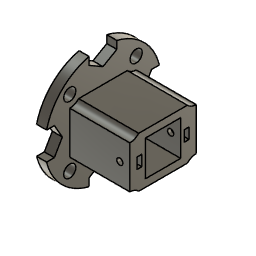
Main_Shredder (Autodesk Fusion 360 archive; units mm, degrees)
design "GearBox_Axle_Conector"
Autodesk Fusion 360 part; units mm, degrees
sketch "Plate" plane through (0, 0, 0) normal (0, 0, 1) x (1, 0, 0)
  circle A0 centre (-28.284, 0) radius 11
  line L0 (0, 0) -> (-28.284, 0) construction
  circle A1 centre (-28.284, 0) radius 4.05
  circle A2 centre (0, -28.284) radius 4.05
  circle A3 centre (0, -28.284) radius 11
  circle A4 centre (28.284, 0) radius 4.05
  circle A5 centre (28.284, 0) radius 11
  circle A6 centre (0, 28.284) radius 4.05
  circle A7 centre (0, 28.284) radius 11
  circle A8 centre (0, 0) radius 39
  dimension "d2" = 22
  dimension "d8" = 28.284
  dimension "d9" = 8.1
  dimension "d11" = 360
  dimension "d42" = 78
  constraint coincident L0.start A8.centre
  constraint coincident A0.centre L0.end
  constraint horizontal L0
  constraint concentric A0 A1
  measures "d2" diameter of A0
  measures "d8" distance of L0.start A0.centre
  measures "d9" diameter of A1
  measures "d42" diameter of A8
extrude "Extrude1" add sketch "Plate" along normal blind 3 contours A0 A8 | A0 A8 | A7 A8 | A7 A8 | A3 A8 | A3 A8 | A5 A8 | A5 A8 makes body 1 at (8.6273, 27.5363, 0) makes body 2 at (36.9113, 0.7477, 3) makes body 3 at (-19.6416, 0.5465, 3) makes body 4 at (8.6273, -27.5363, 3)
extrude "Extrude2" add sketch "Plate" against normal blind 13 bodies 1 2 3 4
chamfer "Chamfer1" distance 5.5 distance2 2.5 4 edges at (-10.2556, 24.3062, 3) (-38.5396, -3.9778, 3) (-10.2556, -32.2618, 3) (18.0284, -3.9778, 3) measured on face at (8.6424, 28.8305, 3) measured on face at (-19.6416, 0.5465, 3) measured on face at (8.6273, -27.5363, 3) measured on face at (36.9113, 0.7477, 3) on bodies 1
extrude "Extrude9" add 4 faces at (-23.2878, 0.2732, 3) (33.2802, 0.2732, 3) (4.9962, 28.5572, 3) (4.9962, -28.0108, 3) along direction (0, 0, 1) blind 1.2 on bodies 1 bodies 1
sketch "BallbearingHole" plane through (0, 0, 0) normal (0, 0, 1) x (1, 0, 0)
  arc A0 (-38.891, -2.9141) -> (-38.891, 2.9141) centre (-28.284, 0) ccw
  arc A1 (-38.891, -2.9141) -> (-2.9141, -38.891) centre (0, 0) ccw
  arc A2 (2.9141, -38.891) -> (-2.9141, -38.891) centre (0, -28.284) ccw
  arc A3 (2.9141, -38.891) -> (38.891, -2.9141) centre (0, 0) ccw
  arc A4 (38.891, 2.9141) -> (38.891, -2.9141) centre (28.284, 0) ccw
  arc A5 (38.891, 2.9141) -> (2.9141, 38.891) centre (0, 0) ccw
  arc A6 (-2.9141, 38.891) -> (2.9141, 38.891) centre (0, 28.284) ccw
  arc A7 (-2.9141, 38.891) -> (-38.891, 2.9141) centre (0, 0) ccw
  circle A8 centre (0, 0) radius 16
  dimension "d22" = 32
  constraint coincident A1.centre A3.centre
  measures "d22" diameter of A8
extrude "Extrude3" cut sketch "BallbearingHole" against normal blind 9.5 contours A8 bodies 1
sketch "BallbearingStandoff" plane through (0, 0, -9.5) normal (0, 0, 1) x (1, 0, 0)
  circle A0 centre (0, 0) radius 16
  circle A1 centre (0, 0) radius 15
  dimension "d25" = -1
extrude "Extrude4" add sketch "BallbearingStandoff" along normal blind 0.5 bodies 1
sketch "Nut" plane through (0, 0, -13) normal (0, 0, -1) x (-1, 0, 0)
  circle A0 centre (-28.284, 0) radius 4.05
  circle A1 centre (0, -28.284) radius 4.05
  circle A2 centre (28.284, 0) radius 4.05
  circle A3 centre (0, 28.284) radius 4.05
  arc A4 (-38.891, 2.9141) -> (-38.891, -2.9141) centre (-28.284, 0) ccw
  arc A5 (-38.891, -2.9141) -> (-2.9141, -38.891) centre (0, 0) ccw
  arc A6 (-2.9141, -38.891) -> (2.9141, -38.891) centre (0, -28.284) ccw
  arc A7 (2.9141, -38.891) -> (38.891, -2.9141) centre (0, 0) ccw
  arc A8 (38.891, -2.9141) -> (38.891, 2.9141) centre (28.284, 0) ccw
  arc A9 (38.891, 2.9141) -> (2.9141, 38.891) centre (0, 0) ccw
  arc A10 (2.9141, 38.891) -> (-2.9141, 38.891) centre (0, 28.284) ccw
  arc A11 (-2.9141, 38.891) -> (-38.891, 2.9141) centre (0, 0) ccw
  line L0 (-32.284, -6.9282) -> (-36.284, 0)
  line L1 (-36.284, 0) -> (-32.284, 6.9282)
  line L2 (-32.284, 6.9282) -> (-24.284, 6.9282)
  line L3 (-24.284, 6.9282) -> (-20.284, 0)
  line L4 (-20.284, 0) -> (-24.284, -6.9282)
  line L5 (-24.284, -6.9282) -> (-32.284, -6.9282)
  line L6 (-20.284, 0) -> (-36.284, 0) construction
  line L7 (-6.9282, -24.284) -> (0, -20.284)
  line L8 (-6.9282, -32.284) -> (-6.9282, -24.284)
  line L9 (0, -36.284) -> (-6.9282, -32.284)
  line L10 (6.9282, -32.284) -> (0, -36.284)
  line L11 (6.9282, -24.284) -> (6.9282, -32.284)
  line L12 (0, -20.284) -> (6.9282, -24.284)
  line L13 (24.284, -6.9282) -> (20.284, 0)
  line L14 (32.284, -6.9282) -> (24.284, -6.9282)
  line L15 (36.284, 0) -> (32.284, -6.9282)
  line L16 (32.284, 6.9282) -> (36.284, 0)
  line L17 (24.284, 6.9282) -> (32.284, 6.9282)
  line L18 (20.284, 0) -> (24.284, 6.9282)
  line L19 (6.9282, 24.284) -> (0, 20.284)
  line L20 (6.9282, 32.284) -> (6.9282, 24.284)
  line L21 (0, 36.284) -> (6.9282, 32.284)
  line L22 (-6.9282, 32.284) -> (0, 36.284)
  line L23 (-6.9282, 24.284) -> (-6.9282, 32.284)
  line L24 (0, 20.284) -> (-6.9282, 24.284)
  dimension "d28" = 120
  dimension "d29" = 120
  dimension "d30" = 120
  dimension "d31" = 8
  dimension "d33" = 360
  constraint equal L0 L1
  constraint equal L1 L2
  constraint equal L2 L3
  constraint equal L3 L4
  constraint equal L4 L5
  constraint horizontal L6
  constraint midpoint A0.centre L6
  measures "d28" angle of L0 L1
  measures "d29" angle of L1 L2
  measures "d30" angle of L2 L3
  measures "d31" distance of L0.end L1.end
  measures "d70" distance of L16.start
  measures "d71" distance of L16.start
extrude "Extrude5" cut sketch "Nut" against normal blind 11.5 contours L0 L1 L2 L3 L4 L5 | L7 L8 L9 L10 L11 L12 | L13 L14 L15 L16 L17 L18 | L19 L20 L21 L22 L23 L24 bodies 1
sketch "Output" plane through (0, 0, -13) normal (0, 0, -1) x (-1, 0, 0)
  line L0 (-24.284, 6.9282) -> (-20.284, 0)
  line L1 (-20.284, 0) -> (-24.284, -6.9282)
  line L2 (-24.284, -6.9282) -> (-32.284, -6.9282)
  line L3 (-32.284, -6.9282) -> (-36.284, 0)
  line L4 (-36.284, 0) -> (-32.284, 6.9282)
  line L5 (-32.284, 6.9282) -> (-24.284, 6.9282)
  line L6 (32.284, -6.9282) -> (24.284, -6.9282)
  line L7 (24.284, -6.9282) -> (20.284, 0)
  line L8 (20.284, 0) -> (24.284, 6.9282)
  line L9 (24.284, 6.9282) -> (32.284, 6.9282)
  line L10 (32.284, 6.9282) -> (36.284, 0)
  line L11 (36.284, 0) -> (32.284, -6.9282)
  line L12 (6.9282, 32.284) -> (6.9282, 24.284)
  line L13 (6.9282, 24.284) -> (0, 20.284)
  line L14 (0, 20.284) -> (-6.9282, 24.284)
  line L15 (-6.9282, 24.284) -> (-6.9282, 32.284)
  line L16 (-6.9282, 32.284) -> (0, 36.284)
  line L17 (0, 36.284) -> (6.9282, 32.284)
  line L18 (-6.9282, -32.284) -> (-6.9282, -24.284)
  line L19 (-6.9282, -24.284) -> (0, -20.284)
  line L20 (0, -20.284) -> (6.9282, -24.284)
  line L21 (6.9282, -24.284) -> (6.9282, -32.284)
  line L22 (6.9282, -32.284) -> (0, -36.284)
  line L23 (0, -36.284) -> (-6.9282, -32.284)
  arc A0 (-38.891, 2.9141) -> (-38.891, -2.9141) centre (-28.284, 0) ccw
  arc A1 (-38.891, -2.9141) -> (-2.9141, -38.891) centre (0, 0) ccw
  arc A2 (-2.9141, -38.891) -> (2.9141, -38.891) centre (0, -28.284) ccw
  arc A3 (2.9141, -38.891) -> (38.891, -2.9141) centre (0, 0) ccw
  arc A4 (38.891, -2.9141) -> (38.891, 2.9141) centre (28.284, 0) ccw
  arc A5 (38.891, 2.9141) -> (2.9141, 38.891) centre (0, 0) ccw
  arc A6 (2.9141, 38.891) -> (-2.9141, 38.891) centre (0, 28.284) ccw
  arc A7 (-2.9141, 38.891) -> (-38.891, 2.9141) centre (0, 0) ccw
  circle A8 centre (0, 0) radius 30
  dimension "d39" = 60
  constraint concentric A1 A8
  measures "d39" diameter of A8
extrude "Extrude6" add sketch "Output" along normal blind 13 contours L0 L1 L2 L5 L6 L7 L8 L9 L12 L13 L14 L15 L18 L19 L20 L21 A8 bodies 1
sketch "Mounting hole Output" plane through (0, 0, -26) normal (0, 0, -1) x (-1, 0, 0)
  line L0 (24.284, 6.9282) -> (29.189, 6.9282)
  arc A0 (29.189, 6.9282) -> (6.9282, 29.189) centre (0, 0) ccw
  line L1 (6.9282, 29.189) -> (6.9282, 24.284)
  line L2 (6.9282, 24.284) -> (0, 20.284)
  line L3 (0, 20.284) -> (-6.9282, 24.284)
  line L4 (-6.9282, 24.284) -> (-6.9282, 29.189)
  arc A1 (-6.9282, 29.189) -> (-29.189, 6.9282) centre (0, 0) ccw
  line L5 (-29.189, 6.9282) -> (-24.284, 6.9282)
  line L6 (-24.284, 6.9282) -> (-20.284, 0)
  line L7 (-20.284, 0) -> (-24.284, -6.9282)
  line L8 (-24.284, -6.9282) -> (-29.189, -6.9282)
  arc A2 (-29.189, -6.9282) -> (-6.9282, -29.189) centre (0, 0) ccw
  line L9 (-6.9282, -29.189) -> (-6.9282, -24.284)
  line L10 (-6.9282, -24.284) -> (0, -20.284)
  line L11 (0, -20.284) -> (6.9282, -24.284)
  line L12 (6.9282, -24.284) -> (6.9282, -29.189)
  arc A3 (6.9282, -29.189) -> (29.189, -6.9282) centre (0, 0) ccw
  line L13 (29.189, -6.9282) -> (24.284, -6.9282)
  line L14 (24.284, -6.9282) -> (20.284, 0)
  line L15 (20.284, 0) -> (24.284, 6.9282)
  circle A4 centre (-16.5817, 16.5817) radius 3.05
  line L16 (0, 0) -> (-16.5817, 16.5817) construction
  line L17 (0, 0) -> (-16.5817, 0) construction
  line L18 (-16.5817, 0) -> (-16.5817, 16.5817) construction
  circle A5 centre (-16.5817, -16.5817) radius 3.05
  circle A6 centre (16.5817, -16.5817) radius 3.05
  circle A7 centre (16.5817, 16.5817) radius 3.05
  dimension "d44" = 6.1
  dimension "d45" = 23.45
  dimension "d47" = 360
  constraint coincident A0.centre A1.centre
  constraint coincident A4.centre L16.end
  constraint horizontal L17
  constraint vertical L18
  constraint equal L17 L18
  measures "d44" diameter of A4
  measures "d45" distance of A0.centre A4.centre
extrude "Extrude7" cut sketch "Mounting hole Output" against normal blind 24.5 contours A4 | A5 | A6 | A7 bodies 1
sketch "OutputHub Nut" plane through (0, 0, 0) normal (0, 0, 1) x (1, 0, 0)
  circle A0 centre (0, 0) radius 16
  arc A1 (-38.891, -2.9141) -> (-38.891, 2.9141) centre (-28.284, 0) ccw
  arc A2 (-38.891, -2.9141) -> (-2.9141, -38.891) centre (0, 0) ccw
  arc A3 (2.9141, -38.891) -> (-2.9141, -38.891) centre (0, -28.284) ccw
  arc A4 (2.9141, -38.891) -> (38.891, -2.9141) centre (0, 0) ccw
  arc A5 (38.891, 2.9141) -> (38.891, -2.9141) centre (28.284, 0) ccw
  arc A6 (38.891, 2.9141) -> (2.9141, 38.891) centre (0, 0) ccw
  arc A7 (-2.9141, 38.891) -> (2.9141, 38.891) centre (0, 28.284) ccw
  arc A8 (-2.9141, 38.891) -> (-38.891, 2.9141) centre (0, 0) ccw
  line L0 (-15.0029, 10.6895) -> (-10.6895, 15.0029)
  line L1 (-10.6895, 15.0029) -> (-12.2683, 20.895)
  line L2 (-12.2683, 20.895) -> (-18.1605, 22.4738)
  line L3 (-18.1605, 22.4738) -> (-22.4738, 18.1605)
  line L4 (-22.4738, 18.1605) -> (-20.895, 12.2683)
  line L5 (-20.895, 12.2683) -> (-15.0029, 10.6895)
  line L6 (0, 0) -> (-12.8462, 12.8462) construction
  line L7 (-12.8462, 12.8462) -> (-12.8462, 0) construction
  line L8 (-12.8462, 0) -> (0, 0) construction
  line L9 (-10.6895, 15.0029) -> (-22.4738, 18.1605) construction
  line L10 (-15.0029, -10.6895) -> (-20.895, -12.2683)
  line L11 (-20.895, -12.2683) -> (-22.4738, -18.1605)
  line L12 (-22.4738, -18.1605) -> (-18.1605, -22.4738)
  line L13 (-18.1605, -22.4738) -> (-12.2683, -20.895)
  line L14 (-12.2683, -20.895) -> (-10.6895, -15.0029)
  line L15 (-10.6895, -15.0029) -> (-15.0029, -10.6895)
  line L16 (10.6895, -15.0029) -> (12.2683, -20.895)
  line L17 (12.2683, -20.895) -> (18.1605, -22.4738)
  line L18 (18.1605, -22.4738) -> (22.4738, -18.1605)
  line L19 (22.4738, -18.1605) -> (20.895, -12.2683)
  line L20 (20.895, -12.2683) -> (15.0029, -10.6895)
  line L21 (15.0029, -10.6895) -> (10.6895, -15.0029)
  line L22 (15.0029, 10.6895) -> (20.895, 12.2683)
  line L23 (20.895, 12.2683) -> (22.4738, 18.1605)
  line L24 (22.4738, 18.1605) -> (18.1605, 22.4738)
  line L25 (18.1605, 22.4738) -> (12.2683, 20.895)
  line L26 (12.2683, 20.895) -> (10.6895, 15.0029)
  line L27 (10.6895, 15.0029) -> (15.0029, 10.6895)
  dimension "d52" = 120
  dimension "d53" = 120
  dimension "d54" = 120
  dimension "d55" = 120
  dimension "d56" = 120
  dimension "d57" = 6.1
  dimension "d59" = 360
  constraint equal L1 L2
  constraint equal L0 L1
  constraint equal L0 L5
  constraint coincident A0.centre A2.centre
  constraint midpoint L0 L6.end
  constraint vertical L7
  constraint perpendicular L7 L8
  constraint equal L7 L8
  constraint perpendicular L0 L6
  measures "d52" angle of L0 L1
  measures "d53" angle of L0 L5
  measures "d54" angle of L4 L5
  measures "d55" angle of L3 L4
  measures "d56" angle of L2 L3
  measures "d57" distance of L2.end L3.end
extrude "Extrude8" cut sketch "OutputHub Nut" against normal blind 5 contours L0 L1 L2 L3 L4 L5 | L10 L11 L12 L13 L14 L15 | L16 L17 L18 L19 L20 L21 | L22 L23 L24 L25 L26 L27 bodies 1
chamfer "Chamfer3" distance 1 angle 45 4 edges at (-21.2132, 21.2132, -26) (21.2132, 21.2132, -26) (21.2132, -21.2132, -26) (-21.2132, -21.2132, -26) on bodies 1
move_body "Move1" bodies 1 to x (0, 0, 1) y (0, 1, 0) z (-1, 0, 0) at (3, 0, 3)
sketch "Sketch8" plane through (29, 0, 0) normal (1, 0, 0) x (0, 1, 0)
  arc A0 (-28.1603, -3.9282) -> (-6.9282, -25.1603) centre (0, 3) ccw
  line L0 (-6.9282, -25.1603) -> (-6.9282, -21.284)
  line L1 (-6.9282, -21.284) -> (0, -17.284)
  line L2 (0, -17.284) -> (6.9282, -21.284)
  line L3 (6.9282, -21.284) -> (6.9282, -25.1603)
  arc A1 (6.9282, -25.1603) -> (28.1603, -3.9282) centre (0, 3) ccw
  line L4 (28.1603, -3.9282) -> (24.284, -3.9282)
  line L5 (24.284, -3.9282) -> (20.284, 3)
  line L6 (20.284, 3) -> (24.284, 9.9282)
  line L7 (24.284, 9.9282) -> (28.1603, 9.9282)
  arc A2 (28.1603, 9.9282) -> (6.9282, 31.1603) centre (0, 3) ccw
  line L8 (6.9282, 31.1603) -> (6.9282, 27.284)
  line L9 (6.9282, 27.284) -> (0, 23.284)
  line L10 (0, 23.284) -> (-6.9282, 27.284)
  line L11 (-6.9282, 27.284) -> (-6.9282, 31.1603)
  arc A3 (-6.9282, 31.1603) -> (-28.1603, 9.9282) centre (0, 3) ccw
  line L12 (-28.1603, 9.9282) -> (-24.284, 9.9282)
  line L13 (-24.284, 9.9282) -> (-20.284, 3)
  line L14 (-20.284, 3) -> (-24.284, -3.9282)
  line L15 (-24.284, -3.9282) -> (-28.1603, -3.9282)
  circle A4 centre (16.5817, -13.5817) radius 3.05
  circle A5 centre (16.5817, 19.5817) radius 3.05
  circle A6 centre (-16.5817, -13.5817) radius 3.05
  circle A7 centre (-16.5817, 19.5817) radius 3.05
  line L16 (0, 23.284) -> (0, -17.284) construction
  line L17 (-20.284, 3) -> (20.284, 3) construction
  line L18 (8.8, -5.8) -> (-8.8, -5.8)
  line L19 (-8.8, -5.8) -> (-8.8, 11.8)
  line L20 (-8.8, 11.8) -> (8.8, 11.8)
  line L21 (8.8, 11.8) -> (8.8, -5.8)
  line L22 (8.8, -5.8) -> (-8.8, 11.8) construction
  line L23 (-8.8, -5.8) -> (8.8, 11.8) construction
  point P0 (0, 3)
  dimension "d66" = 17.6
  dimension "d67" = 17.6
  constraint coincident L9.end L10.start
  constraint coincident L1.end L2.start
  constraint coincident L13.end L14.start
  constraint coincident L5.end L6.start
  constraint horizontal L18
  constraint perpendicular L18 L19
  constraint parallel L18 L20
  constraint parallel L19 L21
  constraint coincident L22 P0
  constraint coincident L23 P0
  constraint coincident P0 A0.centre
  measures "d66" distance of L19.end L20.end
  measures "d67" distance of L18.end L19.end
extrude "Extrude1'" add sketch "Sketch8" along normal blind 5 separate body contours A0 L0 L1 L2 L3 A1 L4 L5 L6 L7 A2 L8 L9 L10 L11 A3 L12 L13 L14 L15 | A4 | A5 | A6 | A7 | L18 L19 L20 L21 makes body 5 in component "Component"
extrude "Extrude2'" cut sketch "Sketch8" along normal blind 13 contours A4 | A5 | A6 | A7 sketch seen with x (1, 0, 0) y (0, 1, 0) z (0, 0, 1) at (-8, 0, 0) bodies 5 in component "Component"
sketch "Sketch9" plane through (42, 0, 0) normal (1, 0, 0) x (0, 1, 0)
  line L0 (-24.284, -3.9282) -> (-28.1603, -3.9282)
  arc A0 (-28.1603, -3.9282) -> (-6.9282, -25.1603) centre (0, 3) ccw
  line L1 (-6.9282, -25.1603) -> (-6.9282, -21.284)
  line L2 (-6.9282, -21.284) -> (0, -17.284)
  line L3 (0, -17.284) -> (6.9282, -21.284)
  line L4 (6.9282, -21.284) -> (6.9282, -25.1603)
  arc A1 (6.9282, -25.1603) -> (28.1603, -3.9282) centre (0, 3) ccw
  line L5 (28.1603, -3.9282) -> (24.284, -3.9282)
  line L6 (24.284, -3.9282) -> (20.284, 3)
  line L7 (20.284, 3) -> (24.284, 9.9282)
  line L8 (24.284, 9.9282) -> (28.1603, 9.9282)
  arc A2 (28.1603, 9.9282) -> (6.9282, 31.1603) centre (0, 3) ccw
  line L9 (6.9282, 31.1603) -> (6.9282, 27.284)
  line L10 (6.9282, 27.284) -> (0, 23.284)
  line L11 (0, 23.284) -> (-6.9282, 27.284)
  line L12 (-6.9282, 27.284) -> (-6.9282, 31.1603)
  arc A3 (-6.9282, 31.1603) -> (-28.1603, 9.9282) centre (0, 3) ccw
  line L13 (-28.1603, 9.9282) -> (-24.284, 9.9282)
  line L14 (-24.284, 9.9282) -> (-20.284, 3)
  line L15 (-20.284, 3) -> (-24.284, -3.9282)
  line L16 (0, 23.284) -> (0, -17.284) construction
  line L17 (-20.284, 3) -> (20.284, 3) construction
  line L18 (8.8, -5.8) -> (-8.8, -5.8)
  line L19 (-8.8, -5.8) -> (-8.8, 11.8)
  line L20 (-8.8, 11.8) -> (8.8, 11.8)
  line L21 (8.8, 11.8) -> (8.8, -5.8)
  line L22 (8.8, -5.8) -> (-8.8, 11.8) construction
  line L23 (-8.8, -5.8) -> (8.8, 11.8) construction
  circle A4 centre (-16.5817, -13.5817) radius 3.05
  circle A5 centre (16.5817, -13.5817) radius 3.05
  circle A6 centre (-16.5817, 19.5817) radius 3.05
  circle A7 centre (16.5817, 19.5817) radius 3.05
  line L24 (-16.5817, -13.5817) -> (-16.5817, -10.5317) construction
  line L25 (16.5817, -13.5817) -> (16.5817, -10.5317) construction
  line L26 (16.5817, 19.5817) -> (16.5817, 16.5317) construction
  line L27 (-16.5817, 19.5817) -> (-16.5817, 16.5317) construction
  line L28 (-16.5817, 16.5317) -> (-16.5817, 15.5317) construction
  line L29 (16.5817, 16.5317) -> (16.5817, 15.5317) construction
  line L30 (16.5817, -10.5317) -> (16.5817, -9.5317) construction
  line L31 (-16.5817, -10.5317) -> (-16.5817, -9.5317) construction
  line L32 (-16.5817, -9.5317) -> (16.5817, -9.5317)
  line L33 (16.5817, 15.5317) -> (16.5817, -9.5317)
  line L34 (-16.5817, 15.5317) -> (16.5817, 15.5317)
  line L35 (-16.5817, -9.5317) -> (-16.5817, 15.5317)
  circle A8 centre (16.5817, -13.5817) radius 6
  circle A9 centre (-16.5817, -13.5817) radius 6
  circle A10 centre (16.5817, 19.5817) radius 6
  circle A11 centre (-16.5817, 19.5817) radius 6
  point P0 (0, 3)
  dimension "d70" = 17.6
  dimension "d71" = 17.6
  dimension "d84" = 1
  dimension "d85" = 1
  dimension "d86" = 1
  dimension "d87" = 1
  dimension "d95" = 12
  dimension "d96" = 12
  dimension "d97" = 12
  dimension "d98" = 12
  constraint coincident L10.end L11.start
  constraint coincident L2.end L3.start
  constraint coincident L14.end L15.start
  constraint coincident L6.end L7.start
  constraint horizontal L18
  constraint perpendicular L18 L19
  constraint parallel L18 L20
  constraint parallel L19 L21
  constraint coincident L22 P0
  constraint coincident L23 P0
  constraint coincident P0 A0.centre
  constraint coincident A4.centre L24.start
  constraint coincident A4 L24.end
  constraint vertical L24
  constraint coincident A5.centre L25.start
  constraint coincident A5 L25.end
  constraint parallel L24 L25
  constraint coincident A7.centre L26.start
  constraint coincident A7 L26.end
  constraint parallel L25 L26
  constraint coincident A6.centre L27.start
  constraint coincident A6 L27.end
  constraint vertical L27
  constraint parallel L27 L28
  constraint parallel L26 L29
  constraint perpendicular L17 L30
  constraint parallel L24 L31
  measures "d70" distance of L19.end L20.end
  measures "d71" distance of L18.end L19.end
  measures "d84" distance of L27.end L28.end
  measures "d85" distance of L24.end L31.end
  measures "d86" distance of L25.end L30.end
  measures "d87" distance of L26.end L29.end
  measures "d95" diameter of A8
  measures "d96" diameter of A9
  measures "d97" diameter of A10
  measures "d98" diameter of A11
extrude "Extrude6'" add sketch "Sketch9" along normal blind 30 contours L32 L35 A9 | L32 L33 L34 L35 A8 A9 A10 A11 | L34 L35 A11 | L32 L33 A8 | L33 L34 A10 sketch seen with x (1, 0, 0) y (0, 1, 0) z (0, 0, 1) at (-8, 0, 0) bodies 5 in component "Component"
sketch "Sketch10" plane through (0, 16.5817, 0) normal (0, 1, 0) x (-1, 0, 0)
  line L0 (-42, -10.5317) -> (-42, 16.5317)
  line L1 (-42, 16.5317) -> (-92, 16.5317)
  line L2 (-92, 16.5317) -> (-92, -10.5317)
  line L3 (-92, -10.5317) -> (-42, -10.5317)
  circle A0 centre (-67, 3) radius 1.55
  line L4 (-42, -9.5317) -> (-42, 15.5317)
  line L5 (-42, 15.5317) -> (-72, 15.5317)
  line L6 (-72, 15.5317) -> (-72, -9.5317)
  line L7 (-72, -9.5317) -> (-42, -9.5317)
  line L8 (-67, 3) -> (-72, 3) construction
  dimension "d78" = 3.1
  constraint coincident A0.centre L8.start
  constraint midpoint L6 L8.end
  measures "d78" diameter of A0
extrude "Extrude7'" cut sketch "Sketch10" against normal blind 35 contours A0 sketch seen with x (1, 0, 0) y (0, 1, 0) z (0, 0, 1) at (-8, 0, 0) bodies 5 in component "Component"
sketch "Sketch11" plane through (0, 0, 15.5317) normal (0, 0, 1) x (-1, 0, 0)
  line L0 (-42, -16.5817) -> (-42, 16.5817)
  line L1 (-42, 16.5817) -> (-92, 16.5817)
  line L2 (-92, 16.5817) -> (-92, -16.5817)
  line L3 (-92, -16.5817) -> (-42, -16.5817)
  line L4 (-66.8436, -16.5817) -> (-66.8436, 18.0661) construction
  line L5 (-92, 0) -> (-82.2253, 0) construction
  circle A0 centre (-66.8436, 0) radius 1.55
  line L6 (-42, -16.5817) -> (-42, 16.5817)
  line L7 (-42, 16.5817) -> (-72, 16.5817)
  line L8 (-72, 16.5817) -> (-72, -16.5817)
  line L9 (-72, -16.5817) -> (-42, -16.5817)
  dimension "d81" = 3.1
  constraint coincident L3 L4.start
  constraint perpendicular L1 L4
  constraint midpoint L2 L5.start
  constraint perpendicular L2 L5
  constraint coincident L5 A0.centre
  constraint coincident L4 A0.centre
  measures "d81" diameter of A0
extrude "Extrude9'" cut sketch "Sketch9" along normal blind 30 contours L32 L35 A9 | L34 L35 A11 | L32 L33 A8 | L33 L34 A10 sketch seen with x (1, 0, 0) y (0, 1, 0) z (0, 0, 1) at (-8, 0, 0) bodies 5 in component "Component"
sketch "Sketch12" plane through (72, 0, 0) normal (1, 0, 0) x (0, 1, 0)
  arc A0 (-16.5817, 13.5817) -> (-12.1547, 15.5317) centre (-16.5817, 19.5817) ccw
  line L0 (-16.5817, 13.5817) -> (-16.5817, -7.5817)
  arc A1 (-12.1547, -9.5317) -> (-16.5817, -7.5817) centre (-16.5817, -13.5817) ccw
  line L1 (-12.1547, -9.5317) -> (12.1547, -9.5317)
  arc A2 (16.5817, -7.5817) -> (12.1547, -9.5317) centre (16.5817, -13.5817) ccw
  line L2 (16.5817, -7.5817) -> (16.5817, 13.5817)
  arc A3 (12.1547, 15.5317) -> (16.5817, 13.5817) centre (16.5817, 19.5817) ccw
  line L3 (12.1547, 15.5317) -> (-12.1547, 15.5317)
  line L4 (-8.8, 11.8) -> (8.8, 11.8)
  line L5 (8.8, 11.8) -> (8.8, -5.8)
  line L6 (8.8, -5.8) -> (-8.8, -5.8)
  line L7 (-8.8, -5.8) -> (-8.8, 11.8)
  line L8 (16.5817, 3) -> (-18.6449, 3) construction
  line L9 (8.8, 3) -> (11.8, 3) construction
  line L10 (-8.8, 3) -> (-11.8, 3) construction
  line L11 (12.98, 5.705) -> (10.62, 5.705)
  line L12 (10.62, 5.705) -> (10.62, 0.295)
  line L13 (10.62, 0.295) -> (12.98, 0.295)
  line L14 (12.98, 0.295) -> (12.98, 5.705)
  line L15 (12.98, 5.705) -> (10.62, 0.295) construction
  line L16 (10.62, 5.705) -> (12.98, 0.295) construction
  line L17 (-10.62, 0.295) -> (-12.98, 0.295)
  line L18 (-12.98, 0.295) -> (-12.98, 5.705)
  line L19 (-12.98, 5.705) -> (-10.62, 5.705)
  line L20 (-10.62, 5.705) -> (-10.62, 0.295)
  line L21 (-10.62, 0.295) -> (-12.98, 5.705) construction
  line L22 (-12.98, 0.295) -> (-10.62, 5.705) construction
  point P0 (11.8, 3)
  point P1 (-11.8, 3)
  dimension "d102" = 3
  dimension "d103" = 3
  dimension "d104" = 2.36
  dimension "d105" = 5.41
  dimension "d109" = 2.36
  dimension "d110" = 5.41
  constraint horizontal L8
  constraint coincident L2 L8.start
  constraint midpoint L2 L8.start
  constraint midpoint L5 L9.start
  constraint perpendicular L5 L9
  constraint midpoint L7 L10.start
  constraint perpendicular L7 L10
  constraint horizontal L11
  constraint perpendicular L11 L12
  constraint parallel L11 L13
  constraint parallel L12 L14
  constraint coincident L15 P0
  constraint coincident L16 P0
  constraint coincident P0 L9.end
  constraint horizontal L17
  constraint perpendicular L17 L18
  constraint parallel L17 L19
  constraint parallel L18 L20
  constraint coincident L21 P1
  constraint coincident L22 P1
  constraint coincident P1 L10.end
  measures "d102" distance of L9.start P0
  measures "d103" distance of L10.start P1
  measures "d104" distance of L12.end L13.end
  measures "d105" distance of L11.end L12.end
  measures "d109" distance of L18.end L19.end
  measures "d110" distance of L17.end L18.end
extrude "Extrude10" cut sketch "Sketch12" against normal blind 7 contours L11 L12 L13 L14 sketch seen with x (1, 0, 0) y (0, 1, 0) z (0, 0, 1) at (-8, 0, 0) bodies 5 in component "Component"
extrude "Extrude11" cut sketch "Sketch12" against normal blind 7 contours L17 L18 L19 L20 sketch seen with x (1, 0, 0) y (0, 1, 0) z (0, 0, 1) at (-8, 0, 0) bodies 5 in component "Component"
component "Component" placed x (1, 0, 0) y (0, 1, 0) z (0, 0, 1) at (8, 0, 0)
equation "PichDiameter_SunGear = 28.284 mm"
equation "PitchDiameter_PlanetGear = 28.284 mm"
equation "GearSpacing = PichDiameter_SunGear / 2 + PitchDiameter_PlanetGear / 2"
equation "M8_Bolt = 8.1 mm"
equation "M8_Nut = 8 mm"
equation "d8 = GearSpacing"
equation "d9 = M8_Bolt"
equation "SmallBallBearingInnerDim = 15 mm"
equation "SmallBallBearingOuterDim = 32 mm"
equation "SmallBallBearingThickness = 9 mm"
equation "d22 = SmallBallBearingOuterDim"
equation "d23 = -SmallBallBearingThickness - 0.5 mm"
equation "d31 = M8_Nut"
equation "LargeBallBearingThickness = 10 mm"
equation "LargeBallBearingOuterDim = 78 mm"
equation "LargeBallBearingInnerDim = 60 mm"
equation "d39 = LargeBallBearingInnerDim"
equation "d40 = LargeBallBearingThickness + 3 mm"
equation "d42 = LargeBallBearingOuterDim"
equation "d44 = M8_BoltAlt"
equation "d45 = LargeBallBearingInnerDim / 2 - M8_Bolt / 2 - 2.5 mm"
equation "M8_BoltAlt = 6.1 mm"
equation "M8_NutAlt = 6 mm"
equation "d57 = M8_BoltAlt"
equation "axle_x_y = 17.6 mm"
equation "d66 = axle_x_y"
equation "d67 = axle_x_y"
equation "d70 = axle_x_y"
equation "d71 = axle_x_y"
equation "conecter_lenght = 30 mm"
equation "conector_screw_size = 3.1 mm"
equation "d78 = conector_screw_size"
equation "d81 = conector_screw_size"
equation "d88 = conecter_lenght"
equation "screw_top = 12 mm"
equation "d95 = screw_top"
equation "d96 = screw_top"
equation "d97 = screw_top"
equation "d98 = screw_top"
equation "mutter_dybde = 5.41 mm"
equation "d104 = mutter_bredde"
equation "d105 = mutter_dybde"
equation "mutter_bredde = 2.36 mm"
equation "d109 = mutter_bredde"
equation "d110 = mutter_dybde"
named bodies: "Output_Hub"
